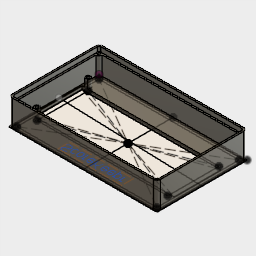
Top_v1 v5 (Autodesk Fusion 360 design; units mm, degrees)
Autodesk Fusion 360 part; units mm, degrees
note: some values were not read from the file. Chosen so that the rebuilt part matches the saved one: that a step has no effect; which face or edge a step refers to. Set by a fixed rule: which sketch regions a step uses.
sketch "Top" plane through (0, 0, 0) normal (0, 1, 0) x (1, 0, 0)
  line L0 (0, 0) -> (128, 0)
  line L1 (128, 0) -> (128, -78)
  line L2 (128, -78) -> (0, -78)
  line L3 (0, -78) -> (0, 0)
  line L4 (0.1275, -34.7956) -> (128, -39)
  line L5 (64, 0) -> (64, -78)
  line L6 (124, -59.3) -> (4, -59.3)
  line L7 (4, -59.3) -> (4, -18.7)
  line L8 (4, -18.7) -> (124, -18.7)
  line L9 (124, -18.7) -> (124, -59.3)
  line L10 (124, -59.3) -> (4, -18.7) construction
  line L11 (4, -59.3) -> (124, -18.7) construction
  line L12 (3.5, -74.5) -> (124.5, -74.5)
  line L13 (124.5, -74.5) -> (124.5, -3.5)
  line L14 (124.5, -3.5) -> (3.5, -3.5)
  line L15 (3.5, -3.5) -> (3.5, -74.5)
  line L16 (3.5, -74.5) -> (124.5, -3.5) construction
  line L17 (124.5, -74.5) -> (3.5, -3.5) construction
  line L18 (120.5, -61.1) -> (7.5, -61.1)
  line L19 (7.5, -61.1) -> (7.5, -16.9)
  line L20 (7.5, -16.9) -> (120.5, -16.9)
  line L21 (120.5, -16.9) -> (120.5, -61.1)
  line L22 (120.5, -61.1) -> (7.5, -16.9) construction
  line L23 (7.5, -61.1) -> (120.5, -16.9) construction
  circle A0 centre (7.5, -16.9) radius 1.15
  circle A1 centre (7.5, -16.9) radius 2.15
  circle A2 centre (120.5, -16.9) radius 1.15
  circle A3 centre (120.5, -16.9) radius 2.15
  circle A4 centre (7.5, -61.1) radius 1.15
  circle A5 centre (7.5, -61.1) radius 2.15
  circle A6 centre (120.5, -61.1) radius 2.15
  circle A7 centre (120.5, -61.1) radius 1.15
  circle A8 centre (3.5, -3.5) radius 1.15
  circle A9 centre (3.5, -3.5) radius 2.15
  circle A10 centre (124.5, -3.5) radius 1.15
  circle A11 centre (124.5, -3.5) radius 2.15
  circle A12 centre (3.5, -74.5) radius 1.15
  circle A13 centre (3.5, -74.5) radius 2.15
  circle A14 centre (124.5, -74.5) radius 1.15
  circle A15 centre (124.5, -74.5) radius 2.15
  line L24 (127, -77) -> (1, -77)
  line L25 (1, -77) -> (1, -1)
  line L26 (1, -1) -> (127, -1)
  line L27 (127, -1) -> (127, -77)
  line L28 (126.5, -76.5) -> (1.5, -76.5)
  line L29 (1.5, -76.5) -> (1.5, -1.5)
  line L30 (1.5, -1.5) -> (126.5, -1.5)
  line L31 (126.5, -1.5) -> (126.5, -76.5)
  line L32 (37.9289, -63.2337) -> (92.7389, -63.2337) construction
  line L33 (92.7389, -63.2337) -> (92.7389, -73.2337) construction
  line L34 (92.7389, -73.2337) -> (37.9289, -73.2337) construction
  line L35 (37.9289, -73.2337) -> (37.9289, -63.2337) construction
  point P0 (64, 0)
  point P1 (128, 0)
  point P2 (64, -39)
  point P3 (64, -39)
  point P4 (64, -39)
  point P5 (64, -39)
  dimension "d8" = 128
  dimension "d9" = 78
  dimension "d13" = 0
  dimension "d16" = 0
  dimension "d17" = 78
  dimension "d20" = 120
  dimension "d21" = 40.6
  dimension "d26" = 71
  dimension "d27" = 121
  dimension "d28" = 113
  dimension "d29" = 44.2
  dimension "d32" = 2.3
  dimension "d33" = 4.3
  dimension "d35" = 2.3
  dimension "d36" = 4.3
  dimension "d37" = 2.3
  dimension "d38" = 4.3
  dimension "d39" = 4.3
  dimension "d40" = 2.3
  dimension "d42" = 2.3
  dimension "d43" = 4.3
  dimension "d44" = 2.3
  dimension "d45" = 4.3
  dimension "d46" = 2.3
  dimension "d47" = 4.3
  dimension "d48" = 2.3
  dimension "d49" = 4.3
  dimension "d103" = 1
  dimension "d104" = 1.5
  measures "d8" distance of L0.start L0.end
  measures "d9" distance of L0.start L2.end
  measures "d20" distance of L7.end L8.end
  measures "d21" distance of L6.end L7.end
  measures "d26" distance of L12.end L13.end
  measures "d27" distance of L13.end L14.end
  measures "d28" distance of L19.end L20.end
  measures "d29" distance of L18.end L19.end
  measures "d32" diameter of A0
  measures "d33" diameter of A1
  measures "d35" diameter of A2
  measures "d36" diameter of A3
  measures "d37" diameter of A4
  measures "d38" diameter of A5
  measures "d39" diameter of A6
  measures "d40" diameter of A7
  measures "d42" diameter of A8
  measures "d43" diameter of A9
  measures "d44" diameter of A10
  measures "d45" diameter of A11
  measures "d46" diameter of A12
  measures "d47" diameter of A13
  measures "d48" diameter of A14
  measures "d49" diameter of A15
extrude "Extrude1" add sketch "Top" along normal blind 23 makes body 1
shell "Shell1" thickness 3 removed faces 1 at (85.3333, 23, 39) on bodies 1
extrude "Extrude2" add sketch "Top" along normal blind 23 separate body contours A9 L30 | L14 L15 A8 A9 L29 L30 | L14 L15 A8 A9 | A9 L29 makes body 2
extrude "Extrude3" cut sketch "Top" along normal blind 23 contours L14 L15 A8 | L14 L15 A8 bodies 1
extrude "Extrude4" cut sketch "Top" along normal blind 3 contours A9 L30 | L14 L15 A8 A9 L29 L30 | L14 L15 A8 A9 | A9 L29 bodies 1 2
extrude "Extrude5" add sketch "Top" along normal blind 23 separate body contours L12 L15 A12 A13 L28 L29 | A13 L28 | A13 L29 | L12 L15 A12 A13 makes body 3
extrude "Extrude6" cut sketch "Top" along normal blind 23 contours L12 L15 A12 | L12 L15 A12 bodies 1
extrude "Extrude7" cut sketch "Top" along normal blind 3 contours L12 L15 A12 A13 L28 L29 | A13 L28 | A13 L29 | L12 L15 A12 A13 bodies 1 3
extrude "Extrude8" add sketch "Top" along normal blind 23 separate body contours A15 L28 | L12 L13 A14 A15 L28 L31 | A15 L31 | L12 L13 A14 A15 makes body 4
extrude "Extrude9" add sketch "Top" along normal blind 23 separate body contours L13 L14 A10 A11 L30 L31 | A11 L30 | L13 L14 A10 A11 | A11 L31 makes body 5
extrude "Extrude10" cut sketch "Top" along normal blind 23 contours L12 L13 A14 | L12 L13 A14 bodies 1
extrude "Extrude11" cut sketch "Top" along normal blind 3 contours A15 L28 | L12 L13 A14 A15 L28 L31 | A15 L31 | L12 L13 A14 A15 bodies 1 4
extrude "Extrude12" cut sketch "Top" along normal blind 23 contours L13 L14 A10 | L13 L14 A10 bodies 1
extrude "Extrude13" cut sketch "Top" along normal blind 3 contours L13 L14 A10 A11 L30 L31 | A11 L30 | L13 L14 A10 A11 | A11 L31 bodies 1 5
extrude "Extrude14" add sketch "Top" along normal blind 10 separate body contours L8 L20 L21 A2 A3 | L8 L20 L21 A2 A3 | L8 L21 A3 | L8 L21 A3 makes body 6
extrude "Extrude15" add sketch "Top" along normal blind 10 separate body contours L6 L18 L21 A6 A7 | L6 L18 L21 A6 A7 | L6 L21 A6 | L6 L21 A6 makes body 7
extrude "Extrude16" add sketch "Top" along normal blind 10 separate body contours L8 L19 L20 A0 A1 | L8 L19 L20 A0 A1 | L8 L19 A1 | L8 L19 A1 makes body 8
extrude "Extrude17" add sketch "Top" along normal blind 10 separate body contours L6 L18 L19 A4 A5 | L6 L18 L19 A4 A5 | L6 L19 A5 | L6 L19 A5 makes body 9
extrude "Extrude18" cut sketch "Top" along normal blind 14.5 contours L4 L5 L8 L21 A3 | L4 L5 L8 L19 A1 | L4 L5 L6 L19 A5 | L4 L5 L6 L21 A6 | L8 L19 A1 | L8 L21 A3 | L6 L21 A6 | L6 L19 A5 picked at (7.6033, -18.9258) picked at (120.3967, -18.9258) picked at (120.3967, -59.0742) picked at (7.6033, -59.0742) bodies 1 6 7 8 9
fillet "Fillet1" radius 3 1 edges at (128, 11.5, 0) on bodies 1
fillet "Fillet2" radius 3 3 edges at (0, 11.5, 0) (0, 11.5, 78) (128, 11.5, 78) on bodies 1
combine "Combine1" operation add target body 1 tool bodies 8 2 9 7 3 5 4 6
extrude "Extrude19" cut sketch "Top" along normal blind 23 contours L4 L6 L9 L21 A6 | L4 L8 L9 L21 A3 | L8 L21 A3 | L6 L21 A6 | L6 L21 A6 picked at (120.6033, -18.9258) bodies 1
extrude "Extrude20" cut sketch "Top" along normal blind 23 contours L4 L7 L8 L19 A1 | L8 L19 A1 | L4 L6 L7 L19 A5 | L6 L19 A5 picked at (7.3967, -18.9258) picked at (7.3967, -59.0742) bodies 1
sketch "Top Lip" plane through (0, 23, 0) normal (0, 1, 0) x (-1, 0, 0)
  line L0 (-122.4089, 75) -> (-5.5911, 75)
  arc A0 (-5.5911, 75) -> (-3, 72.4089) centre (-3.5, 74.5) ccw
  line L1 (-3, 72.4089) -> (-3, 5.5911)
  arc A1 (-3, 5.5911) -> (-5.5911, 3) centre (-3.5, 3.5) ccw
  line L2 (-5.5911, 3) -> (-122.4089, 3)
  arc A2 (-122.4089, 3) -> (-125, 5.5911) centre (-124.5, 3.5) ccw
  line L3 (-125, 5.5911) -> (-125, 72.4089)
  arc A3 (-125, 72.4089) -> (-122.4089, 75) centre (-124.5, 74.5) ccw
  circle A4 centre (-124.5, 74.5) radius 1.15
  circle A5 centre (-124.5, 3.5) radius 1.15
  circle A6 centre (-3.5, 74.5) radius 1.15
  arc A7 (-125, 78) -> (-128, 75) centre (-125, 75) ccw
  line L4 (-128, 75) -> (-128, 3)
  arc A8 (-128, 3) -> (-125, 0) centre (-125, 3) ccw
  line L5 (-125, 0) -> (-3, 0)
  arc A9 (-3, 0) -> (0, 3) centre (-3, 3) ccw
  line L6 (0, 3) -> (0, 75)
  arc A10 (0, 75) -> (-3, 78) centre (-3, 75) ccw
  line L7 (-3, 78) -> (-125, 78)
  circle A11 centre (-3.5, 3.5) radius 1.15
  arc A12 (-125, 77) -> (-127, 75) centre (-125, 75) ccw
  line L8 (-127, 75) -> (-127, 3)
  arc A13 (-127, 3) -> (-125, 1) centre (-125, 3) ccw
  line L9 (-125, 1) -> (-3, 1)
  arc A14 (-3, 1) -> (-1, 3) centre (-3, 3) ccw
  line L10 (-1, 3) -> (-1, 75)
  arc A15 (-1, 75) -> (-3, 77) centre (-3, 75) ccw
  line L11 (-3, 77) -> (-125, 77)
  line L12 (-3, 76.5) -> (-125, 76.5)
  arc A16 (-125, 76.5) -> (-126.5, 75) centre (-125, 75) ccw
  line L13 (-126.5, 75) -> (-126.5, 3)
  arc A17 (-126.5, 3) -> (-125, 1.5) centre (-125, 3) ccw
  line L14 (-125, 1.5) -> (-3, 1.5)
  arc A18 (-3, 1.5) -> (-1.5, 3) centre (-3, 3) ccw
  line L15 (-1.5, 3) -> (-1.5, 75)
  arc A19 (-1.5, 75) -> (-3, 76.5) centre (-3, 75) ccw
  dimension "d99" = 1
  dimension "d100" = 1.5
extrude "Extrude23" cut sketch "Top Lip" against normal blind 4 contours L12 A16 L13 A17 L14 A18 L15 A19 bodies 1
extrude "Extrude30" [no effect]
extrude "Extrude33" [suppressed]
sketch "Sketch8" plane through (0, 0, 0) normal (0, 1, 0) x (1, 0, 0)
  line L0 (21.5535, -9.8303) -> (19.8137, -10.1538)
  spline S0 degree 3 poles (19.8137, -10.1538) (19.7713, -10.1618) (19.725, -10.2016) (19.7107, -10.2424) knots 0 0 0 0 1 1 1 1
  line L1 (19.7107, -10.2424) -> (19.1774, -11.4866)
  spline S1 degree 3 poles (19.1774, -11.4866) (19.1575, -11.525) (19.1613, -11.5854) (19.1859, -11.6211) knots 0 0 0 0 1 1 1 1
  line L2 (19.1859, -11.6211) -> (20.1995, -13.0986)
  spline S2 degree 3 poles (20.1995, -13.0986) (20.2238, -13.1341) (20.219, -13.1882) (20.1884, -13.2188) knots 0 0 0 0 1 1 1 1
  line L3 (20.1884, -13.2188) -> (18.9223, -14.4849)
  spline S3 degree 3 poles (18.9223, -14.4849) (18.8918, -14.5155) (18.8378, -14.5204) (18.8022, -14.496) knots 0 0 0 0 1 1 1 1
  line L4 (18.8022, -14.496) -> (17.2989, -13.4643)
  spline S4 degree 3 poles (17.2989, -13.4643) (17.2633, -13.4399) (17.2023, -13.4355) (17.1637, -13.4546) knots 0 0 0 0 1 1 1 1
  line L5 (17.1637, -13.4546) -> (15.9576, -13.9483)
  spline S5 degree 3 poles (15.9576, -13.9483) (15.9167, -13.9618) (15.8768, -14.0077) (15.8687, -14.0501) knots 0 0 0 0 1 1 1 1
  line L6 (15.8687, -14.0501) -> (15.5338, -15.8496)
  spline S6 degree 3 poles (15.5338, -15.8496) (15.5259, -15.892) (15.4841, -15.9267) (15.441, -15.9267) knots 0 0 0 0 1 1 1 1
  line L7 (15.441, -15.9267) -> (13.6503, -15.9267)
  spline S7 degree 3 poles (13.6503, -15.9267) (13.6072, -15.9267) (13.5654, -15.892) (13.5576, -15.8496) knots 0 0 0 0 1 1 1 1
  line L8 (13.5576, -15.8496) -> (13.2227, -14.0501)
  spline S8 degree 3 poles (13.2227, -14.0501) (13.2147, -14.0077) (13.1749, -13.9618) (13.1338, -13.9483) knots 0 0 0 0 1 1 1 1
  line L9 (13.1338, -13.9483) -> (11.9276, -13.4546)
  spline S9 degree 3 poles (11.9276, -13.4546) (11.8889, -13.4355) (11.8279, -13.4399) (11.7925, -13.4643) knots 0 0 0 0 1 1 1 1
  line L10 (11.7925, -13.4643) -> (10.2892, -14.496)
  spline S10 degree 3 poles (10.2892, -14.496) (10.2535, -14.5204) (10.1995, -14.5155) (10.169, -14.4849) knots 0 0 0 0 1 1 1 1
  line L11 (10.169, -14.4849) -> (8.9028, -13.2188)
  spline S11 degree 3 poles (8.9028, -13.2188) (8.8723, -13.1882) (8.8672, -13.1341) (8.8917, -13.0986) knots 0 0 0 0 1 1 1 1
  line L12 (8.8917, -13.0986) -> (9.9055, -11.6211)
  spline S12 degree 3 poles (9.9055, -11.6211) (9.9298, -11.5854) (9.9336, -11.525) (9.9138, -11.4866) knots 0 0 0 0 1 1 1 1
  line L13 (9.9138, -11.4866) -> (9.3804, -10.2424)
  spline S13 degree 3 poles (9.3804, -10.2424) (9.3662, -10.2016) (9.32, -10.1618) (9.2774, -10.1538) knots 0 0 0 0 1 1 1 1
  line L14 (9.2774, -10.1538) -> (7.5377, -9.8303)
  spline S14 degree 3 poles (7.5377, -9.8303) (7.4952, -9.8223) (7.4606, -9.7806) (7.4606, -9.7374) knots 0 0 0 0 1 1 1 1
  line L15 (7.4606, -9.7374) -> (7.4607, -7.9468)
  spline S15 degree 3 poles (7.4607, -7.9468) (7.4607, -7.9036) (7.4954, -7.8616) (7.5379, -7.8539) knots 0 0 0 0 1 1 1 1
  line L16 (7.5379, -7.8539) -> (9.2349, -7.5381)
  spline S16 degree 3 poles (9.2349, -7.5381) (9.2773, -7.5303) (9.3227, -7.49) (9.3356, -7.4489) knots 0 0 0 0 1 1 1 1
  line L17 (9.3356, -7.4489) -> (9.8654, -6.1254)
  spline S17 degree 3 poles (9.8654, -6.1254) (9.8844, -6.0866) (9.8799, -6.0258) (9.8554, -5.9903) knots 0 0 0 0 1 1 1 1
  line L18 (9.8554, -5.9903) -> (8.8915, -4.5855)
  spline S18 degree 3 poles (8.8915, -4.5855) (8.8671, -4.55) (8.8721, -4.4958) (8.9026, -4.4652) knots 0 0 0 0 1 1 1 1
  line L19 (8.9026, -4.4652) -> (10.1689, -3.1991)
  spline S19 degree 3 poles (10.1689, -3.1991) (10.1994, -3.1687) (10.2534, -3.1638) (10.2891, -3.188) knots 0 0 0 0 1 1 1 1
  line L20 (10.2891, -3.188) -> (11.669, -4.1351)
  spline S20 degree 3 poles (11.669, -4.1351) (11.7045, -4.1594) (11.7641, -4.1614) (11.8012, -4.1397) knots 0 0 0 0 1 1 1 1
  line L21 (11.8012, -4.1397) -> (12.4098, -3.8147)
  spline S21 degree 3 poles (12.4098, -3.8147) (12.4483, -3.7951) (12.4933, -3.8117) (12.5098, -3.8516) knots 0 0 0 0 1 1 1 1
  line L22 (12.5098, -3.8516) -> (13.7646, -6.8834)
  spline S22 degree 3 poles (13.7646, -6.8834) (13.7812, -6.9233) (13.7646, -6.9742) (13.7277, -6.9967) knots 0 0 0 0 1 1 1 1
  line L23 (13.7277, -6.9967) -> (13.5754, -7.09)
  spline S23 degree 3 poles (13.5754, -7.09) (13.5473, -7.1071) (13.5091, -7.1366) (13.4791, -7.1637) knots 0 0 0 0 1 1 1 1
  spline S24 degree 3 poles (13.4791, -7.1637) (12.9297, -7.5155) (12.5653, -8.131) (12.5653, -8.8318) knots 0 0 0 0 1 1 1 1
  spline S25 degree 3 poles (12.5653, -8.8318) (12.5653, -9.9255) (13.4519, -10.812) (14.5455, -10.812) knots 0 0 0 0 1 1 1 1
  spline S26 degree 3 poles (14.5455, -10.812) (15.6391, -10.812) (16.5256, -9.9255) (16.5256, -8.8318) knots 0 0 0 0 1 1 1 1
  spline S27 degree 3 poles (16.5256, -8.8318) (16.5256, -8.131) (16.1613, -7.5155) (15.6118, -7.1637) knots 0 0 0 0 1 1 1 1
  spline S28 degree 3 poles (15.6118, -7.1637) (15.582, -7.1366) (15.5437, -7.1071) (15.5157, -7.09) knots 0 0 0 0 1 1 1 1
  line L24 (15.5157, -7.09) -> (15.3634, -6.9967)
  spline S29 degree 3 poles (15.3634, -6.9967) (15.3268, -6.9742) (15.31, -6.9233) (15.3266, -6.8834) knots 0 0 0 0 1 1 1 1
  line L25 (15.3266, -6.8834) -> (16.5812, -3.8515)
  spline S30 degree 3 poles (16.5812, -3.8515) (16.5977, -3.8116) (16.6426, -3.7951) (16.6812, -3.8146) knots 0 0 0 0 1 1 1 1
  line L26 (16.6812, -3.8146) -> (17.2898, -4.1396)
  spline S31 degree 3 poles (17.2898, -4.1396) (17.327, -4.1612) (17.3865, -4.1594) (17.4221, -4.135) knots 0 0 0 0 1 1 1 1
  line L27 (17.4221, -4.135) -> (18.802, -3.1879)
  spline S32 degree 3 poles (18.802, -3.1879) (18.8376, -3.1637) (18.8918, -3.1686) (18.9221, -3.199) knots 0 0 0 0 1 1 1 1
  line L28 (18.9221, -3.199) -> (20.1884, -4.4651)
  spline S33 degree 3 poles (20.1884, -4.4651) (20.219, -4.4957) (20.224, -4.5499) (20.1995, -4.5854) knots 0 0 0 0 1 1 1 1
  line L29 (20.1995, -4.5854) -> (19.2355, -5.9902)
  spline S34 degree 3 poles (19.2355, -5.9902) (19.2112, -6.0257) (19.2066, -6.0865) (19.2256, -6.1253) knots 0 0 0 0 1 1 1 1
  line L30 (19.2256, -6.1253) -> (19.7554, -7.4488)
  spline S35 degree 3 poles (19.7554, -7.4488) (19.7684, -7.4899) (19.8135, -7.5302) (19.856, -7.538) knots 0 0 0 0 1 1 1 1
  line L31 (19.856, -7.538) -> (21.553, -7.8538)
  spline S36 degree 3 poles (21.553, -7.8538) (21.5954, -7.8615) (21.6302, -7.9035) (21.6302, -7.9467) knots 0 0 0 0 1 1 1 1
  line L32 (21.6302, -7.9467) -> (21.6304, -9.7373)
  spline S37 degree 3 poles (21.6304, -9.7373) (21.6305, -9.7806) (21.5958, -9.8223) (21.5535, -9.8303) knots 0 0 0 0 1 1 1 1
extrude "Extrude34" [suppressed]
extrude "Extrude25" [suppressed]
extrude "Extrude21" [suppressed]
equation "caseheight = 75 mm"
equation "lcdholewidth = 112 mm"
equation "lcdholeheight = 45 mm"
equation "lcdveroffset = 1.8 mm"
equation "casewidth = 125 mm"
equation "shell = 3 mm"
equation "d8 = casewidth + shell"
equation "d9 = caseheight + shell"
equation "d12 = ( casewidth + shell )"
equation "d17 = caseheight + shell"
equation "lcdwidth = 120 mm"
equation "lcdheight = 40.6 mm"
equation "d20 = lcdwidth"
equation "d21 = lcdheight"
equation "lcdhoroffest = 3.5 mm"
equation "caseholdoffset = 2 mm"
equation "d26 = caseheight - ( caseholdoffset * 2 )"
equation "d27 = casewidth - ( caseholdoffset * 2 )"
equation "d28 = lcdwidth - ( lcdhoroffest * 2 )"
equation "d29 = lcdheight + ( lcdveroffset * 2 )"
equation "lcdpostwall = 2 mm"
equation "lcdposthole = 2.3 mm"
equation "d32 = lcdposthole"
equation "d33 = lcdposthole + lcdpostwall"
equation "caseradius = 3 mm"
equation "d35 = lcdposthole"
equation "d36 = lcdposthole + lcdpostwall"
equation "d37 = lcdposthole"
equation "d38 = lcdposthole + lcdpostwall"
equation "d39 = lcdposthole + lcdpostwall"
equation "d40 = lcdposthole"
equation "casedepth = 23 mm"
equation "d42 = lcdposthole"
equation "d43 = lcdpostwall + lcdposthole"
equation "d44 = lcdposthole"
equation "d45 = lcdposthole + lcdpostwall"
equation "d46 = lcdposthole"
equation "d47 = lcdpostwall + lcdposthole"
equation "d48 = lcdposthole"
equation "d49 = lcdposthole + lcdpostwall"
equation "d50 = casedepth"
equation "d52 = shell"
equation "d53 = casedepth"
equation "d55 = casedepth"
equation "d59 = casedepth"
equation "d61 = casedepth"
equation "d65 = casedepth"
equation "d67 = casedepth"
equation "d69 = casedepth"
equation "d73 = casedepth"
equation "holeheight = 10 mm"
equation "d78 = holeheight"
equation "d80 = holeheight"
equation "d82 = holeheight"
equation "d84 = holeheight"
equation "d88 = caseradius"
equation "d89 = caseradius"
equation "switchwidth = 12.5 mm"
equation "switchheight = 19 mm"
equation "d92 = casedepth"
equation "d94 = casedepth"
equation "lipwidth = 1 mm"
equation "lipdepth = 4 mm"
equation "lipclearance = 0.5 mm"
equation "d101 = -lipdepth"
equation "bottomdepth = 30 mm"
equation "d134 = -lipdepth"
equation "d142 = bottomdepth"
equation "d162 = -( bottomdepth - shell )"
equation "bottompostheight = 7 mm"
named bodies: "Top"
